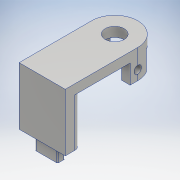
# Autodesk Inventor part: Casing Attachment MH
Saved by Autodesk Inventor 2018 (Build 220112000, 112)
## iProperties
Created: 2018-01-24
Part Number: Casing Attachment MH
Material: Aluminum 6061
Document SubType Name: Modeling
Designer: Moochster
Density: 2.7 g/cm^3
Appearance: Aluminum - Flat
Author: Moochster
Autodesk Inventor part; units mm, degrees
ref_plane "YZ Plane" through (0, 0, 0) normal (1, 0, 0) x (0, 1, 0)
ref_plane "XZ Plane" through (0, 0, 0) normal (0, 1, 0) x (-1, 0, 0)
ref_plane "XY Plane" through (0, 0, 0) normal (0, 0, 1) x (1, 0, 0)
sketch "Sketch1" plane through (0, 0, 0) normal (0, 0, 1) x (1, 0, 0)
  line L0 (-12, 0) -> (12, 0)
  line L1 (12, 0) -> (12, 37.7)
  arc A0 (12, 37.7) -> (-12, 37.7) centre (0, 37.7) ccw
  line L2 (-12, 37.7) -> (-12, 0)
  circle A1 centre (0, 37.7) radius 4.925
  line L3 (12, 8) -> (-12, 8)
  line L4 (6, 6) -> (-6, 6) construction
  line L5 (-6, 6) -> (-6, 2) construction
  line L6 (-6, 2) -> (6, 2) construction
  line L7 (6, 2) -> (6, 6) construction
  line L8 (-5.84, 2.16) -> (-5.84, 5.84)
  line L9 (-5.84, 5.84) -> (5.84, 5.84)
  line L10 (5.84, 5.84) -> (5.84, 2.16)
  line L11 (5.84, 2.16) -> (-5.84, 2.16)
  point P0 (0, 0)
  point P1 (0, 0)
  point P2 (0, 2)
  dimension "d0" = 24
  dimension "d1" = 37.7
  dimension "d2" = 9.85
  dimension "d5" = 8
  dimension "d6" = 2
  dimension "d7" = 4
  dimension "d8" = 12
  dimension "d9" = 0.16
  constraints: 24 end point, 4 parallel, 4 perpendicular, 3 coincident, 2 centre point, 2 horizontal, 2 midpoint, 2 point on circle, 2 point on line, 2 tangent, 1 vertical, 1 vertical alignment, 3 other
  measures "d0" distance of L0.start L0.end
  measures "d1" distance from line of L0 A0.centre
  measures "d2" diameter of A1
  measures "d5" distance between parallel lines of L0 L3
  measures "d6" distance between parallel lines of L0 L6
  measures "d7" distance of L4.end L5.end
  measures "d8" distance of L5.end L6.end
  measures "d9" distance between parallel lines of L5 L8
extrude "Extrusion1" add sketch "Sketch1" along normal blind 5 contours L2 L3 L1 L0 | L2 A0 L1 L3 | L8 L9 L10 L11
extrude "Extrusion2" add sketch "Sketch1" against normal blind 25 contours L2 L3 L1 L0 | L8 L9 L10 L11
sketch "Sketch3" plane through (0, 0, -25) normal (0, 0, -1) x (-1, 0, 0)
  line L0 (-5.84, 5.84) -> (-5.84, 2.16) projected
  line L1 (5.84, 5.84) -> (-5.84, 5.84) projected
  line L2 (5.84, 2.16) -> (5.84, 5.84) projected
  line L3 (-5.84, 2.16) -> (5.84, 2.16) projected
  point P0 (0, 0)
extrude "Extrusion3" add sketch "Sketch3" along normal blind 7.5
fillet "Fillet1" radius 0.5 4 edges at (-5.84, 5.84, -28.75) (-5.84, 2.16, -28.75) (5.84, 2.16, -28.75) (5.84, 5.84, -28.75)
fillet "Fillet2" radius 3 2 edges at (-12, 8, -12.5) (12, 8, -12.5)
sketch "Sketch4" plane through (0, 0, 0) normal (0, 0, -1) x (-1, 0, 0)
  line L0 (0, 41.7) -> (17.7659, 41.7) construction
  line L1 (17.7659, 41.7) -> (17.7659, 33.7) construction
  line L2 (17.7659, 33.7) -> (12, 33.7) construction
  line L3 (0, 33.7) -> (0, 41.7) construction
  arc A0 (12, 37.7) -> (-12, 37.7) centre (0, 37.7) ccw projected
  line L4 (12, 37.7) -> (12, 0) projected
  arc A1 (7.5, 37.7) -> (6.3443, 41.7) centre (0, 37.7) ccw
  line L5 (7.5, 37.7) -> (7.5, 33.7)
  line L6 (6.3443, 41.7) -> (10.1509, 44.1)
  line L7 (7.5, 33.7) -> (0, 33.7) construction
  line L8 (12, 33.7) -> (7.5, 33.7)
  arc A2 (6.3443, 41.7) -> (-7.5, 37.7) centre (0, 37.7) ccw construction
  line L9 (7.5, 33.7) -> (7.5, 0) construction
  point P0 (0, 0)
  point P1 (17.7659, 37.7)
  dimension "d16" = 8
  dimension "d17" = 4.5
  constraints: 18 end point, 5 point on circle, 4 parallel, 2 centre point, 2 line through centre, 2 midpoint, 2 point on line, 2 tangent, 1 horizontal, 1 horizontal alignment, 1 perpendicular
  measures "d16" distance of L0.end L1.end
  measures "d17" distance between parallel lines of L4 L5
extrude "Extrusion4" add sketch "Sketch4" along normal blind 10
mirror "Mirror1" about plane through (0, 0, 0) normal (1, 0, 0) of "Extrusion4"
sketch "Sketch5" plane through (0, 0, 0) normal (1, 0, 0) x (0, 1, 0)
  line L0 (32.775, 5) -> (42.625, 5) projected
  line L1 (42.625, 0) -> (32.775, 0) projected
  circle A0 centre (37.7, -5) radius 2
  line L2 (41.7, 0) -> (41.7, -10) projected
  point P0 (0, 0)
  point P1 (41.7, -5)
  point P2 (37.7, 5)
  dimension "d20" = 4
  constraints: 2 midpoint, 1 centre point, 1 horizontal alignment, 1 vertical alignment
  measures "d20" diameter of A0
extrude "Extrusion5" cut sketch "Sketch5" along normal through all both and the other way through all
body "Solid1"
